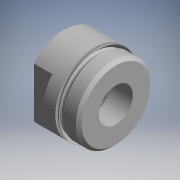
# Autodesk Inventor part: 040000_rear_head
Saved by Autodesk Inventor 2017.3 (Build 213256000, 256)
## iProperties
Part Number: 040000_rear_head
Material: Generic
Catalog Web Link: www.cadenas.de
Description: Rear Head-Original Line - Standard Air Cylinders
Vendor: BIMBA
Document SubType Name: Modeling
Designer: partserver
Manufacturer: BIMBA
Mass: 3.07277 g
Surface Area: 18.9574 cm^2
Volume: 3.07277 cm^3
Density: 1 g/cm^3
Appearance: PSOLRGB-211-211-211
Category: PARTsolutions
Company: BIMBA
Title: 040000_rear_head
Author: Cadenas PARTsolutions
Comments: Original Line - Standard Air Cylinders
PSOL_IDENT_0: {$CADENAS_DATA\23d-libs\bimba\bimba_brand\bimba_imperial\bimba_full_line\original_line_cylinders\sta
PSOL_IDENT_1: ndard_air_cylinders\rear_head.prj},237 {VTYP=3D},{NB=040000_rear_head},{LINA=040000_rear_head},{NN=R
PSOL_IDENT_2: ear Head},{DATE=19.01.2022 10:19:37},{GEOMDATE=11.01.2022 11:41:00},{VERSION=},{LINEID=40},{WBVAR=MN
PSOL_IDENT_3: T,ACTING,DER,Q,T1,T2,T3,T4,TRIM,Y,K,MB,CUSH,FBON},{WBNUMERIC=TRIM,MB,CUSH}  {NB=040000_rear_head},{L
PSOL_IDENT_4: INA=040000_rear_head},{KT=DUMMY},{PN=040000},{BORE=0.75000},{BOREPN=04},{MNT=},{MNTALG='' , 'Front N
PSOL_IDENT_5: ose' , 'P' , 'Rear Pivot' , 'LS' , 'Built-in Valve LS' , 'DX' , 'Double End' , 'BR' , 'Rear Block' ,
PSOL_IDENT_6: 'BRT' , 'Rear Trunnion' , 'A' , 'Adjustable Stroke'},{ACTING=},{ACTINGALG= '' , 'Single Acting' , '
PSOL_IDENT_7: R' , 'Reverse/Double Acting'   },{DER=},{DERALG= '' , 'Standard' },{Q=},{T1=},{T2=},{T3=},{T4=},{TRI
PSOL_IDENT_8: M=0},{Y=},{K=},{KALG= '', 'without K', 'K', 'with K' },{MB=0},{A1=0.5310},{A1N=0.5310},{A1P=1.5940},
PSOL_IDENT_9: {A1B=1.0940},{A1S=1.2190},{A2=0.219},{A2N=0.2190},{A3=0.0300},{D1=0.8050},{D1N=0.8050},{D1P=0.8625},
PSOL_IDENT_10: {D1B=0.8325},{D2=0.7615},{C1=0.0300},{C2=0.0000},{NDM=0.4050},{TAB=NPT},{NDMDP=0.3020},{D3=0.3440},{
PSOL_IDENT_11: A4=0.1880},{A5=0.6200},{D4=0.0000},{A6=0.0000},{A7=0.7500},{A8=0.1250},{D5=0.8170},{D6=0.3120},{A9=0
PSOL_IDENT_12: .8440},{NDM2=0.6250},{TAB2=UNF},{C11=0.0300},{C22=0.0000},{C33=0.0227},{C44=0.0300},{A10=0.3725},{A1
PSOL_IDENT_13: 1=0.0000},{NDM3=0.4050},{NDM3N=0.4050},{NDM3B=0.4050},{TAB3=NPT},{TAB3N=NPT},{TAB3B=NPT},{A12=0.688}
PSOL_IDENT_14: ,{A12N=0.6880},{A12B=0.6560},{A13=1.3120},{D7=0.2520},{D8=0.6225},{A14=0.0940},{A15=0.0855},{D9=0.53
PSOL_IDENT_15: 85},{R1=0.0350},{X1=0.0000},{X2=0.0000},{CX=0.0000},{CC=0.0000},{CON=0},{S1=1.0000},{DB=0.2500},{X1B=
PSOL_IDENT_16: 0.4380},{X2B=0.0310},{A8B=0.1250},{A9B=0.8750},{MODEL=1},{NDM4=0.1900},{TAB4=UNF},{NDM4DP=0.2500},{B
PSOL_IDENT_17: C=1.0000},{B1=0.7150},{B2=0.5000},{B3=0.5000},{ON=0},{ON2=1},{G1=0.1250},{G2=0.5620},{G3=0.6250},{G4=
PSOL_IDENT_18: 0.6250},{GD=0.2520},{G5=0.6250},{G6=0.3725},{RON=0},{H1=1.1175},{H2=0.8170},{H3=0.1250},{H4=0.0350},
PSOL_IDENT_19: {H5=0.9420},{H6=0.5620},{F=0.4380},{PNUT=0.0000},{CUSH=0},{CC11=0.238},{CC111=0.2380},{CC22=0.2750},
PSOL_IDENT_20: {CC33=0.1950},{CC44=0.3700},{CC55=0.5350},{CD1=0.1900},{CD2=0.1500},{CD3=0.0725},{CNDM3=0.1380},{CTA
PSOL_IDENT_21: B3=UNF},{OLEN=0.5310},{OD=0.3455},{STDIS=0.1560},{STDIS1=0.1560},{BUSHCON=D-3543},{BUSHL=0.3700},{FB
PSOL_IDENT_22: ON=0},{LCD=0.0000}
NB: 040000_rear_head
NN: Rear Head
NT: Original Line - Standard Air Cylinders
NBSYN: $PN._rear_head
LINA: 040000_rear_head
CATALOG: Bimba Products
PN: 040000
BORE: 0.75
BOREPN: 04
MNT: Front Nose
MNTALG: '' , 'Front Nose' , 'P' , 'Rear Pivot' , 'LS' , 'Built-in Valve LS' , 'DX' , 'Double End' , 'BR' , 'Rear Block' , 'BRT' , 'Rear Trunnion' , 'A' , 'Adjustable Stroke'
ACTING: Single Acting
DER: Standard
Q: Without Side Ported Rear Head
T1: without T1
T2: without T2
T3: without T3
T4: without T4
TRIM: 0
Y: without Pivot Bushing
K: without K
MB: 0
A1N: 0.531
A1P: 1.594
A1B: 1.094
A1S: 1.219
A2N: 0.219
A3: 0.03
D1N: 0.805
D1P: 0.8625
D1B: 0.8325
D2: 0.7615
C1: 0.03
C2: 0
TAB: NPT
NDMDP: 0.302
D3: 0.344
A4: 0.188
A5: 0.62
D4: 0
A6: 0
A7: 0.75
A8: 0.125
D5: 0.817
D6: 0.312
A9: 0.844
NDM2: 0.625
TAB2: UNF
C11: 0.03
C22: 0
C33: 0.0227
C44: 0.03
A10: 0.3725
A11: 0
NDM3N: 0.405
NDM3B: 0.405
TAB3N: NPT
TAB3B: NPT
A12N: 0.688
A12B: 0.656
A13: 1.312
D7: 0.252
D8: 0.6225
A14: 0.094
A15: 0.0855
D9: 0.5385
R1: 0.035
X1: 0
X2: 0
CX: 0
CC: 0
S1: 1
DB: 0.25
X1B: 0.438
X2B: 0.031
A8B: 0.125
A9B: 0.875
NDM4: 0.19
TAB4: UNF
NDM4DP: 0.25
BC: 1
B1: 0.715
B2: 0.5
B3: 0.5
G1: 0.125
G2: 0.562
G3: 0.625
G4: 0.625
GD: 0.252
G5: 0.625
G6: 0.3725
H2: 0.817
H3: 0.125
F: 0.438
CUSH: 0
CC111: 0.238
CC22: 0.275
CC33: 0.195
CC44: 0.37
CC55: 0.535
CD1: 0.19
CD2: 0.15
CD3: 0.0725
CNDM3: 0.138
CTAB3: UNF
OD: 0.3455
STDIS1: 0.156
BUSHCON: D-3543
BUSHL: 0.37
FBON: 0
LCD: 0
SUPPLIER: BIMBA
ARTICLENO: 040000_rear_head
BOMINFO: 040000_rear_head
CREATOR: CADENAS GmbH
Autodesk Inventor part; units mm, degrees
ref_plane "YZ Plane" through (0, 0, 0) normal (1, 0, 0) x (0, 1, 0)
ref_plane "XZ Plane" through (0, 0, 0) normal (0, 1, 0) x (-1, 0, 0)
ref_plane "XY Plane" through (0, 0, 0) normal (0, 0, 1) x (1, 0, 0)
sketch "Sketch_1" plane through (0, 0, 0) normal (0, 0, 1) x (1, 0, 0)
  line L0 (13.4874, 0) -> (0, 0)
  line L1 (0, 0) -> (0, 8.9091)
  line L2 (0, 8.9091) -> (0.762, 9.671)
  line L3 (0.762, 9.671) -> (4.0386, 9.671)
  line L4 (4.0386, 9.671) -> (4.8006, 8.9091)
  line L5 (4.8006, 8.9091) -> (5.5626, 8.9091)
  line L6 (5.5626, 8.9091) -> (5.5626, 10.2235)
  line L7 (5.5626, 10.2235) -> (13.4874, 10.2235)
  line L8 (13.4874, 10.2235) -> (13.4874, 0)
  line L9 (13.4874, 0) -> (0, 0)
  constraints: 20 end point
revolve "Revolution1" add sketch "Sketch_1" angle 360 about axis through (13.4874, 0, 0) along (1, 0, 0)
sketch "Sketch_6" plane through (0, 0, 0) normal (0, 0, 1) x (1, 0, 0)
  line L0 (13.4874, 0) -> (0, 0)
  line L1 (0, 0) -> (0, 4.3688)
  line L2 (0, 4.3688) -> (-1.5889, 4.3688)
  line L3 (-1.5889, 4.3688) -> (12.8524, 4.8197)
  line L4 (12.8524, 4.8197) -> (13.4874, 5.4547)
  line L5 (13.4874, 5.4547) -> (13.4874, 0)
  line L6 (13.4874, 0) -> (0, 0)
  constraints: 14 end point
revolve "Revolution2" cut sketch "Sketch_6" angle 360 about axis through (13.4874, 0, 0) along (1, 0, 0)
thread "Thread1" size "1/8" designation "1/8 - 27 NPT" standard "NPT" length 7.0392
sketch "Sketch_5" plane through (13.4874, 0, 0) normal (1, 0, 0) x (0, 0, -1)
  line L0 (-40.894, -20.447) -> (40.894, -20.447)
  line L1 (40.894, -20.447) -> (40.894, 20.447)
  line L2 (40.894, 20.447) -> (-40.894, 20.447)
  line L3 (-40.894, 20.447) -> (-40.894, -20.447)
  line L4 (-20.447, -7.874) -> (20.447, -7.874)
  line L5 (20.447, -7.874) -> (20.447, 7.874)
  line L6 (20.447, 7.874) -> (-20.447, 7.874)
  line L7 (-20.447, 7.874) -> (-20.447, -7.874)
  constraints: 16 end point
extrude "Extrusion1" cut sketch "Sketch_5" against normal blind 4.7752
sketch "Sketch_24" plane through (0, 0, 0) normal (0, 0, 1) x (1, 0, 0)
  line L0 (5.5626, 0) -> (4.8006, 0)
  line L1 (4.6479, 10.2235) -> (4.6479, 10.1393)
  line L2 (4.6479, 10.1393) -> (5.4401, 9.3472)
  arc A0 (5.4401, 9.1676) -> (5.4401, 9.3472) centre (5.3503, 9.2574) ccw
  line L3 (5.4401, 9.1676) -> (5.1816, 8.9091)
  line L4 (5.1816, 8.9091) -> (4.8006, 8.9091)
  line L5 (4.8006, 8.9091) -> (4.8006, 8.655)
  line L6 (4.8006, 8.655) -> (5.5626, 8.655)
  line L7 (5.5626, 8.655) -> (5.5626, 9.512)
  line L8 (5.5626, 9.512) -> (4.8511, 10.2235)
  line L9 (4.8511, 10.2235) -> (4.6479, 10.2235)
  constraints: 20 end point, 2 point on circle, 1 centre point
revolve "Revolution3" add sketch "Sketch_24" angle 360 about axis through (5.5626, 0, 0) along (1, 0, 0)
ref_plane "cut1_XY" through (13.4874, 7.874, 0) normal (1, 0, 0) x (0, 0, -1)
ref_plane "cut1_YZ" through (13.4874, 7.874, 0) normal (0, 0, -1) x (0, 1, 0)
ref_plane "cut1_ZX" through (13.4874, 7.874, 0) normal (0, 1, 0) x (1, 0, 0)
ref_plane "cut2_XY" through (13.4874, -7.874, 0) normal (1, 0, 0) x (0, 0, -1)
ref_plane "cut2_YZ" through (13.4874, -7.874, 0) normal (0, 0, -1) x (0, 1, 0)
ref_plane "cut2_ZX" through (13.4874, -7.874, 0) normal (0, 1, 0) x (1, 0, 0)
ref_plane "cutf1_XY" through (13.4874, 0, 0) normal (0, 0, 1) x (1, 0, 0)
ref_plane "cutf1_YZ" through (13.4874, 0, 0) normal (1, 0, 0) x (0, 1, 0)
ref_plane "cutf1_ZX" through (13.4874, 0, 0) normal (0, 1, 0) x (0, 0, 1)
ref_plane "cutf2_XY" through (8.7122, 0, 0) normal (0, 0, 1) x (1, 0, 0)
ref_plane "cutf2_YZ" through (8.7122, 0, 0) normal (1, 0, 0) x (0, 1, 0)
ref_plane "cutf2_ZX" through (8.7122, 0, 0) normal (0, 1, 0) x (0, 0, 1)
ref_plane "lovra_XY" through (13.4874, 0, 0) normal (1, 0, 0) x (0, 1, 0)
ref_plane "lovra_YZ" through (13.4874, 0, 0) normal (0, 1, 0) x (0, 0, 1)
ref_plane "lovra_ZX" through (13.4874, 0, 0) normal (0, 0, 1) x (1, 0, 0)
ref_plane "lovra1_XY" through (8.7122, 0, 0) normal (1, 0, 0) x (0, 0, -1)
ref_plane "lovra1_YZ" through (8.7122, 0, 0) normal (0, 0, -1) x (0, 1, 0)
ref_plane "lovra1_ZX" through (8.7122, 0, 0) normal (0, 1, 0) x (1, 0, 0)
ref_plane "lovra2_XY" through (8.7122, 7.874, 0) normal (1, 0, 0) x (0, 0, -1)
ref_plane "lovra2_YZ" through (8.7122, 7.874, 0) normal (0, 0, -1) x (0, 1, 0)
ref_plane "lovra2_ZX" through (8.7122, 7.874, 0) normal (0, 1, 0) x (1, 0, 0)
ref_plane "lovra21_XY" through (0, 0, 5.2705) normal (1, 0, 0) x (0, 0, -1)
ref_plane "lovra21_YZ" through (0, 0, 5.2705) normal (0, 0, -1) x (0, 1, 0)
ref_plane "lovra21_ZX" through (0, 0, 5.2705) normal (0, 1, 0) x (1, 0, 0)
ref_plane "lovra22_XY" through (0, 0, -5.2705) normal (1, 0, 0) x (0, 0, -1)
ref_plane "lovra22_YZ" through (0, 0, -5.2705) normal (0, 0, -1) x (0, 1, 0)
ref_plane "lovra22_ZX" through (0, 0, -5.2705) normal (0, 1, 0) x (1, 0, 0)
ref_plane "lovra3_XY" through (8.7122, -7.874, 0) normal (1, 0, 0) x (0, 0, -1)
ref_plane "lovra3_YZ" through (8.7122, -7.874, 0) normal (0, 0, -1) x (0, 1, 0)
ref_plane "lovra3_ZX" through (8.7122, -7.874, 0) normal (0, 1, 0) x (1, 0, 0)
ref_plane "olen_XY" through (13.4874, 0, 0) normal (1, 0, 0) x (0, 0, -1)
ref_plane "olen_YZ" through (13.4874, 0, 0) normal (0, 0, -1) x (0, 1, 0)
ref_plane "olen_ZX" through (13.4874, 0, 0) normal (0, 1, 0) x (1, 0, 0)
ref_plane "to_mounting_bracket_XY" through (24.6126, 0, 0) normal (1, 0, 0) x (0, 0, -1)
ref_plane "to_mounting_bracket_YZ" through (24.6126, 0, 0) normal (0, 0, -1) x (0, 1, 0)
ref_plane "to_mounting_bracket_ZX" through (24.6126, 0, 0) normal (0, 1, 0) x (1, 0, 0)
ref_plane "to_nut_XY" through (0, 0, 0) normal (1, 0, 0) x (0, 0, -1)
ref_plane "to_nut_YZ" through (0, 0, 0) normal (0, 0, -1) x (0, 1, 0)
ref_plane "to_nut_ZX" through (0, 0, 0) normal (0, 1, 0) x (1, 0, 0)
ref_plane "to_pin_XY" through (33.3248, 0, 0) normal (0, 1, 0) x (1, 0, 0)
ref_plane "to_pin_YZ" through (33.3248, 0, 0) normal (1, 0, 0) x (0, 0, -1)
ref_plane "to_pin_ZX" through (33.3248, 0, 0) normal (0, 0, -1) x (0, 1, 0)
ref_plane "to_pin_1_XY" through (33.3248, 0, 0) normal (0, 0, 1) x (1, 0, 0)
ref_plane "to_pin_1_YZ" through (33.3248, 0, 0) normal (1, 0, 0) x (0, 1, 0)
ref_plane "to_pin_1_ZX" through (33.3248, 0, 0) normal (0, 1, 0) x (0, 0, 1)
ref_plane "to_pin_r_XY" through (33.3248, 0, 0) normal (0, 0, 1) x (1, 0, 0)
ref_plane "to_pin_r_YZ" through (33.3248, 0, 0) normal (1, 0, 0) x (0, 1, 0)
ref_plane "to_pin_r_ZX" through (33.3248, 0, 0) normal (0, 1, 0) x (0, 0, 1)
ref_plane "to_screw_XY" through (17.4752, 2.032, -6.0452) normal (0, 1, 0) x (1, 0, 0)
ref_plane "to_screw_YZ" through (17.4752, 2.032, -6.0452) normal (1, 0, 0) x (0, 0, -1)
ref_plane "to_screw_ZX" through (17.4752, 2.032, -6.0452) normal (0, 0, -1) x (0, 1, 0)
ref_plane "to_tube_XY" through (4.8006, 0, 0) normal (1, 0, 0) x (0, 0, -1)
ref_plane "to_tube_YZ" through (4.8006, 0, 0) normal (0, 0, -1) x (0, 1, 0)
ref_plane "to_tube_ZX" through (4.8006, 0, 0) normal (0, 1, 0) x (1, 0, 0)
body "Solid1"
